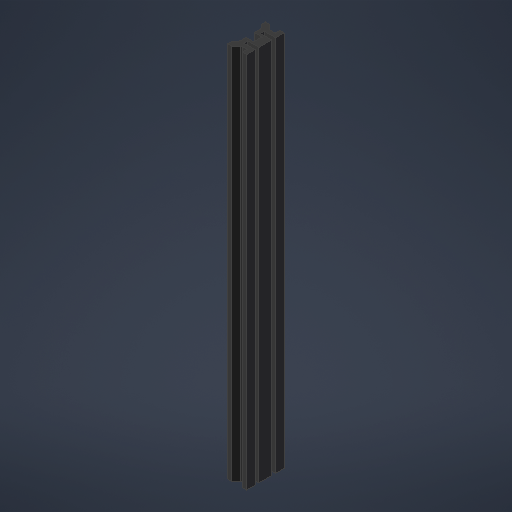
# Autodesk Inventor part: rale
Saved by Autodesk Inventor 2026 (Build 300175050, 175E)
## iProperties
Created: 2025-07-08
Part Number: rale
Material: 一般
Document SubType Name: Modeling
Designer: jin20
Density: 1 g/cm^3
Appearance: 既定
Author: jin20
Autodesk Inventor part; units mm, degrees
ref_plane "YZ Plane" through (0, 0, 0) normal (1, 0, 0) x (0, 1, 0)
ref_plane "XZ Plane" through (0, 0, 0) normal (0, 1, 0) x (-1, 0, 0)
ref_plane "XY Plane" through (0, 0, 0) normal (0, 0, 1) x (1, 0, 0)
sketch "スケッチ1" plane through (0, 0, 0) normal (0, 1, 0) x (-1, 0, 0)
  line L0 (192.8837, 109.7192) -> (992.8837, 109.7192)
  line L1 (722.1337, 89.7192) -> (722.1337, 99.7192)
  line L2 (596.1337, 89.7192) -> (596.1337, 99.7192)
  line L3 (113.1292, 213.8732) -> (123.1292, 213.8732)
  line L4 (663.6337, 89.7192) -> (663.6337, 99.7192)
  line L5 (661.3837, 109.7192) -> (661.3837, 99.7192)
  line L6 (113.1292, 205.1232) -> (103.2292, 205.1232)
  line L7 (724.3837, 99.7192) -> (724.3837, 109.7192)
  line L8 (103.2292, 211.6232) -> (113.1292, 211.6232)
  line L9 (861.3837, 99.7192) -> (861.3837, 109.7192)
  line L10 (113.1292, 202.8732) -> (123.1292, 202.8732)
  line L11 (661.3837, 99.7192) -> (724.3837, 99.7192)
  line L12 (261.3837, 99.7192) -> (324.3837, 99.7192)
  line L13 (223.3837, 99.7192) -> (223.3837, 109.7192)
  line L14 (212.3837, 109.7192) -> (212.3837, 99.7192)
  line L15 (208.3837, 99.7192) -> (208.3837, 109.7192)
  line L16 (197.3837, 109.7192) -> (197.3837, 99.7192)
  line L17 (113.1292, 213.8732) -> (113.1292, 202.8732)
  line L18 (199.6337, 99.7192) -> (199.6337, 89.7192)
  line L19 (206.1337, 89.7192) -> (206.1337, 99.7192)
  line L20 (197.3837, 99.7192) -> (208.3837, 99.7192)
  line L21 (212.3837, 99.7192) -> (223.3837, 99.7192)
  line L22 (214.6337, 99.7192) -> (214.6337, 89.7192)
  line L23 (221.1337, 89.7192) -> (221.1337, 99.7192)
  line L24 (261.3837, 99.7192) -> (261.3837, 109.7192)
  line L25 (263.6337, 89.7192) -> (263.6337, 99.7192)
  line L26 (461.3837, 99.7192) -> (524.3837, 99.7192)
  line L27 (324.3837, 99.7192) -> (324.3837, 109.7192)
  line L28 (322.1337, 89.7192) -> (322.1337, 99.7192)
  line L29 (398.3837, 99.7192) -> (398.3837, 109.7192)
  line L30 (387.3837, 99.7192) -> (387.3837, 109.7192)
  line L31 (398.3837, 99.7192) -> (387.3837, 99.7192)
  line L32 (389.6337, 99.7192) -> (389.6337, 89.7192)
  line L33 (396.1337, 89.7192) -> (396.1337, 99.7192)
  line L34 (461.3837, 109.7192) -> (461.3837, 99.7192)
  line L35 (463.6337, 99.7192) -> (463.6337, 89.7192)
  line L36 (524.3837, 99.7192) -> (524.3837, 109.7192)
  line L37 (522.1337, 89.7192) -> (522.1337, 99.7192)
  line L38 (587.3837, 99.7192) -> (587.3837, 109.7192)
  line L39 (598.3837, 99.7192) -> (598.3837, 109.7192)
  line L40 (587.3837, 99.7192) -> (598.3837, 99.7192)
  line L41 (589.6337, 99.7192) -> (589.6337, 89.7192)
  line L42 (798.3837, 99.7192) -> (787.3837, 99.7192)
  line L43 (787.3837, 99.7192) -> (787.3837, 109.7192)
  line L44 (798.3837, 99.7192) -> (798.3837, 109.7192)
  line L45 (789.6337, 99.7192) -> (789.6337, 89.7192)
  line L46 (796.1337, 89.7192) -> (796.1337, 99.7192)
  line L47 (924.3837, 99.7192) -> (861.3837, 99.7192)
  line L48 (863.6337, 89.7192) -> (863.6337, 99.7192)
  line L49 (924.3837, 109.7192) -> (924.3837, 99.7192)
  line L50 (922.1337, 89.7192) -> (922.1337, 99.7192)
  line L51 (962.3837, 99.7192) -> (962.3837, 109.7192)
  line L52 (973.3837, 109.7192) -> (973.3837, 99.7192)
  line L53 (973.3837, 99.7192) -> (962.3837, 99.7192)
  line L54 (964.6337, 99.7192) -> (964.6337, 89.7192)
  line L55 (971.1337, 89.7192) -> (971.1337, 99.7192)
  line L56 (977.3837, 99.7192) -> (977.3837, 109.7192)
  line L57 (988.3837, 109.7192) -> (988.3837, 99.7192)
  line L58 (988.3837, 99.7192) -> (977.3837, 99.7192)
  line L59 (986.1337, 99.7192) -> (986.1337, 89.7192)
  line L60 (979.6337, 89.7192) -> (979.6337, 99.7192)
  line L61 (103.2292, 199.8732) -> (103.2292, 216.8732)
  line L62 (123.1292, 221.1423) -> (123.1292, 195.6041)
  line L63 (118.1292, 194.7732) -> (118.1292, 199.8732)
  line L64 (103.1292, 194.7732) -> (118.1292, 194.7732)
  line L65 (114.8297, 189.7732) -> (108.8292, 189.7732)
  line L66 (103.1292, 183.3732) -> (103.1292, 194.7732)
  line L67 (108.8292, 183.3732) -> (103.1292, 183.3732)
  line L68 (108.8292, 189.7732) -> (108.8292, 183.3732)
  arc A0 (116.951, 188.8945) -> (114.8297, 189.7732) centre (114.8297, 186.7732) ccw
  line L69 (122.4724, 183.3732) -> (116.951, 188.8945)
  arc A1 (123.1292, 195.6041) -> (124.2422, 192.9171) centre (126.9292, 195.6041) ccw
  line L70 (118.1292, 199.8732) -> (103.1292, 199.8732)
  line L71 (116.951, 227.8519) -> (122.4724, 233.3732)
  line L72 (108.8292, 233.3732) -> (108.8292, 226.9732)
  line L73 (103.1292, 221.9732) -> (103.1292, 233.3732)
  line L74 (108.8292, 226.9732) -> (114.8297, 226.9732)
  line L75 (103.1292, 216.8732) -> (118.1292, 216.8732)
  arc A2 (114.8297, 226.9732) -> (116.951, 227.8519) centre (114.8297, 229.9732) ccw
  line L76 (118.1292, 216.8732) -> (118.1292, 221.9732)
  arc A3 (124.2422, 223.8293) -> (123.1292, 221.1423) centre (126.9292, 221.1423) ccw
  line L77 (103.1292, 233.3732) -> (108.8292, 233.3732)
  line L78 (128.1292, 189.03) -> (128.1292, 183.3732)
  line L79 (128.1292, 233.3732) -> (128.1292, 227.7163)
  circle A4 centre (217.8837, 208.3732) radius 5.5
  circle A5 centre (202.8837, 208.3732) radius 5.5
  line L80 (192.8837, 183.3732) -> (192.8837, 233.3732)
  circle A6 centre (202.8837, 208.3732) radius 3.25
  circle A7 centre (217.8837, 208.3732) radius 3.25
  arc A8 (266.8837, 213.8732) -> (266.8837, 202.8732) centre (266.8837, 208.3732) ccw
  arc A9 (266.8837, 211.6232) -> (266.8837, 205.1232) centre (266.8837, 208.3732) ccw
  arc A10 (466.8837, 211.6232) -> (466.8837, 205.1232) centre (466.8837, 208.3732) ccw
  arc A11 (466.8837, 213.8732) -> (466.8837, 202.8732) centre (466.8837, 208.3732) ccw
  arc A12 (318.8837, 202.8732) -> (318.8837, 213.8732) centre (318.8837, 208.3732) ccw
  arc A13 (318.8837, 205.1232) -> (318.8837, 211.6232) centre (318.8837, 208.3732) ccw
  line L81 (118.1292, 221.9732) -> (103.1292, 221.9732)
  circle A14 centre (392.8837, 208.3732) radius 3.25
  line L82 (518.8837, 202.8732) -> (466.8837, 202.8732)
  line L83 (466.8837, 213.8732) -> (518.8837, 213.8732)
  line L84 (518.8837, 205.1232) -> (466.8837, 205.1232)
  line L85 (466.8837, 211.6232) -> (518.8837, 211.6232)
  arc A15 (518.8837, 202.8732) -> (518.8837, 213.8732) centre (518.8837, 208.3732) ccw
  arc A16 (518.8837, 205.1232) -> (518.8837, 211.6232) centre (518.8837, 208.3732) ccw
  circle A17 centre (592.8837, 208.3732) radius 5.5
  circle A18 centre (592.8837, 208.3732) radius 3.25
  line L86 (992.8837, 227.7592) -> (192.8837, 227.7592)
  line L87 (192.8837, 222.6392) -> (992.8837, 222.6392)
  line L88 (992.8837, 194.1072) -> (192.8837, 194.1072)
  line L89 (192.8837, 188.9872) -> (992.8837, 188.9872)
  line L90 (992.8837, 183.3732) -> (192.8837, 183.3732)
  line L91 (192.8837, 233.3732) -> (992.8837, 233.3732)
  circle A19 centre (392.8837, 208.3732) radius 5.5
  line L92 (992.8837, 109.0041) -> (192.8837, 109.0041)
  line L93 (192.8837, 95.4192) -> (992.8837, 95.4192)
  line L94 (992.8837, 114.7192) -> (192.8837, 114.7192)
  line L95 (192.8837, 89.7192) -> (992.8837, 89.7192)
  line L96 (192.8837, 114.7192) -> (192.8837, 89.7192)
  line L97 (318.8837, 211.6232) -> (266.8837, 211.6232)
  line L98 (266.8837, 205.1232) -> (318.8837, 205.1232)
  line L99 (318.8837, 213.8732) -> (266.8837, 213.8732)
  line L100 (266.8837, 202.8732) -> (318.8837, 202.8732)
  line L101 (122.4724, 233.3732) -> (128.1292, 233.3732)
  line L102 (992.8837, 89.7192) -> (992.8837, 114.7192)
  line L103 (128.1292, 183.3732) -> (122.4724, 183.3732)
  line L104 (124.2422, 192.9171) -> (128.1292, 189.03)
  line L105 (128.1292, 227.7163) -> (124.2422, 223.8293)
  line L106 (718.8837, 202.8732) -> (666.8837, 202.8732)
  line L107 (666.8837, 213.8732) -> (718.8837, 213.8732)
  line L108 (718.8837, 205.1232) -> (666.8837, 205.1232)
  line L109 (666.8837, 211.6232) -> (718.8837, 211.6232)
  arc A20 (666.8837, 213.8732) -> (666.8837, 202.8732) centre (666.8837, 208.3732) ccw
  arc A21 (666.8837, 211.6232) -> (666.8837, 205.1232) centre (666.8837, 208.3732) ccw
  arc A22 (718.8837, 202.8732) -> (718.8837, 213.8732) centre (718.8837, 208.3732) ccw
  arc A23 (718.8837, 205.1232) -> (718.8837, 211.6232) centre (718.8837, 208.3732) ccw
  circle A24 centre (792.8837, 208.3732) radius 5.5
  circle A25 centre (792.8837, 208.3732) radius 3.25
  line L110 (918.8837, 202.8732) -> (866.8837, 202.8732)
  line L111 (866.8837, 213.8732) -> (918.8837, 213.8732)
  line L112 (918.8837, 205.1232) -> (866.8837, 205.1232)
  line L113 (866.8837, 211.6232) -> (918.8837, 211.6232)
  arc A26 (866.8837, 213.8732) -> (866.8837, 202.8732) centre (866.8837, 208.3732) ccw
  arc A27 (866.8837, 211.6232) -> (866.8837, 205.1232) centre (866.8837, 208.3732) ccw
  arc A28 (918.8837, 202.8732) -> (918.8837, 213.8732) centre (918.8837, 208.3732) ccw
  arc A29 (918.8837, 205.1232) -> (918.8837, 211.6232) centre (918.8837, 208.3732) ccw
  circle A30 centre (967.8837, 208.3732) radius 5.5
  circle A31 centre (967.8837, 208.3732) radius 3.25
  line L114 (992.8837, 233.3732) -> (992.8837, 183.3732)
  circle A32 centre (982.8837, 208.3732) radius 5.5
  circle A33 centre (982.8837, 208.3732) radius 3.25
  line L115 (217.8837, 202.3244) -> (217.8837, 214.422)
  line L116 (124.452, 208.3732) -> (101.9808, 208.3732)
  line L117 (202.8837, 88.8748) -> (202.8837, 110.4834)
  line L118 (967.8837, 110.2411) -> (967.8837, 88.9362)
  line L119 (866.8837, 202.3361) -> (866.8837, 214.4103)
  line L120 (993.8179, 208.3732) -> (191.2647, 208.3732)
  line L121 (592.8837, 202.2218) -> (592.8837, 214.5246)
  line L122 (892.8837, 214.6548) -> (892.8837, 202.0916)
  line L123 (918.8837, 202.3658) -> (918.8837, 214.3806)
  line L124 (866.8837, 101.8736) -> (866.8837, 88.958)
  line L125 (392.8837, 202.2198) -> (392.8837, 214.5266)
  line L126 (967.8837, 214.5927) -> (967.8837, 202.1537)
  line L127 (202.8837, 214.3834) -> (202.8837, 202.363)
  line L128 (982.8837, 88.8748) -> (982.8837, 110.4834)
  line L129 (982.8837, 202.188) -> (982.8837, 214.5584)
  line L130 (918.8837, 101.732) -> (918.8837, 88.7983)
  line L131 (792.8837, 214.5493) -> (792.8837, 202.1971)
  line L132 (892.8837, 88.3376) -> (892.8837, 110.5911)
  line L133 (666.8837, 202.3361) -> (666.8837, 214.4103)
  line L134 (692.8837, 214.8254) -> (692.8837, 202.2622)
  line L135 (718.8837, 202.2968) -> (718.8837, 214.3116)
  line L136 (266.8837, 202.3361) -> (266.8837, 214.4103)
  line L137 (292.8837, 214.6548) -> (292.8837, 202.0916)
  line L138 (318.8837, 202.3658) -> (318.8837, 214.3806)
  line L139 (466.8837, 202.3361) -> (466.8837, 214.4103)
  line L140 (492.8837, 214.6548) -> (492.8837, 202.0916)
  line L141 (518.8837, 202.3658) -> (518.8837, 214.3806)
  line L142 (466.8837, 101.8736) -> (466.8837, 88.958)
  line L143 (518.8837, 101.732) -> (518.8837, 88.7983)
  line L144 (492.8837, 88.3376) -> (492.8837, 110.5911)
  line L145 (266.8837, 101.8736) -> (266.8837, 88.958)
  line L146 (318.8837, 101.732) -> (318.8837, 88.7983)
  line L147 (292.8837, 88.3376) -> (292.8837, 110.5911)
  line L148 (666.8837, 101.8736) -> (666.8837, 88.958)
  line L149 (718.8837, 101.732) -> (718.8837, 88.7983)
  line L150 (692.8837, 88.3376) -> (692.8837, 110.5911)
  line L151 (792.8837, 88.8748) -> (792.8837, 110.4834)
  line L152 (592.8837, 88.8748) -> (592.8837, 110.4834)
  line L153 (392.8837, 88.8748) -> (392.8837, 110.4834)
  line L154 (217.8837, 88.8748) -> (217.8837, 110.4834)
  point P0 (0, 0)
  point P1 (560.6317, 21.4808)
  point P2 (124.2422, 223.8293)
  point P3 (116.951, 227.8519)
  point P4 (124.2422, 192.9171)
  constraints: 310 end point, 40 point on circle, 34 centre point, 1 other
extrude "押し出し1" add sketch "スケッチ1" along normal blind 500 contours L17 L8 L61 L75 L76 L81 L73 L77 L72 L74 A2 L71 L101 L79 L105 A3 L62 L3 | L17 L116 L61 L8 | L17 L6 L61 L116 | L62 A1 L104 L78 L103 L69 A0 L65 L68 L67 L66 L64 L63 L70 L61 L6 L17 L10
